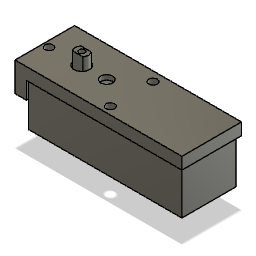
Moteur arduino v15 (Autodesk Fusion 360 design; units mm, degrees)
Autodesk Fusion 360 part; units mm, degrees
sketch "Esquisse1" plane through (0, 0, 0) normal (0, 1, 0) x (1, 0, 0)
  line L0 (0, 0) -> (64, 0)
  line L1 (64, 0) -> (64, 22.3)
  line L2 (64, 22.3) -> (0, 22.3)
  line L3 (0, 22.3) -> (0, 0)
  line L4 (0, 22.3) -> (10.9, 22.3)
  line L5 (10.9, 22.3) -> (10.9, 11.15)
  line L6 (10.9, 11.15) -> (0, 11.15)
  line L7 (0, 11.15) -> (0, 22.3)
  circle A0 centre (10.9, 11.15) radius 2.9
  line L8 (0, 22.3) -> (31.8, 22.3)
  line L9 (31.8, 22.3) -> (31.8, 20.1)
  line L10 (31.8, 20.1) -> (0, 20.1)
  line L11 (0, 20.1) -> (0, 22.3)
  circle A1 centre (31.8, 20.1) radius 1.8
  line L12 (0, 0) -> (31.8, 0)
  line L13 (31.8, 0) -> (31.8, 2.2)
  line L14 (31.8, 2.2) -> (0, 2.2)
  line L15 (0, 2.2) -> (0, 0)
  circle A2 centre (31.8, 2.2) radius 1.8
  dimension "d1" = 64
  dimension "d2" = 22.3
  dimension "d3" = 10.9
  dimension "d4" = 11.15
  dimension "d5" = 5.8
  dimension "d8" = 31.8
  dimension "d9" = 2.2
  dimension "d10" = 3.6
  dimension "d11" = 31.8
  dimension "d12" = 2.2
  dimension "d13" = 3.6
  constraint horizontal L0
  constraint vertical L1
  constraint horizontal L2
  constraint vertical L3
  constraint coincident L0.start L3.end
  constraint horizontal L4
  constraint vertical L5
  constraint horizontal L6
  constraint vertical L7
  constraint coincident L5.end L6.start
  constraint horizontal L8
  constraint vertical L9
  constraint horizontal L10
  constraint vertical L11
  constraint coincident L9.end L10.start
  constraint horizontal L12
  constraint vertical L13
  constraint horizontal L14
  constraint vertical L15
  constraint coincident L13.end L14.start
  measures "d1" distance of L0.start L0.end
  measures "d2" distance of L0.start L2.end
  measures "d3" distance of L2.end L4.end
  measures "d4" distance of L2.end L6.end
  measures "d5" diameter of A0
  measures "d8" distance of L2.end L8.end
  measures "d9" distance of L2.end L10.end
  measures "d10" diameter of A1
  measures "d11" distance of L0.start L12.end
  measures "d12" distance of L0.start L14.end
  measures "d13" diameter of A2
extrude "Extrusion1" add sketch "Esquisse1" along normal blind 19 contours L0 L3 L12 L13 L14 L15 A2 | L0 L1 L2 L3 L5 L6 A0 L9 L10 A1 L13 L14 A2 | L3 L5 L6 L7 A0 L10 | L2 L3 L4 L5 L7 L8 L10 L11 | L2 L5 L8 L9 L10 A1 makes body 1
sketch "Esquisse2" plane through (0, 0, 0) normal (-1, 0, 0) x (0, 0, 1)
  line L0 (-22.3, 0) -> (0, 0)
  line L1 (0, 0) -> (0, 19)
  line L2 (0, 19) -> (-22.3, 19)
  line L3 (-22.3, 19) -> (-22.3, 0)
  line L4 (-22.3, 19) -> (-13.3, 19)
  line L5 (-13.3, 19) -> (-13.3, 11)
  line L6 (-13.3, 11) -> (-22.3, 11)
  line L7 (-22.3, 11) -> (-22.3, 19)
  line L8 (-13.3, 11) -> (-8.3, 11)
  line L9 (-8.3, 11) -> (-8.3, 8)
  line L10 (-8.3, 8) -> (-13.3, 8)
  line L11 (-13.3, 8) -> (-13.3, 11)
  dimension "d14" = 9
  dimension "d15" = 8
  dimension "d16" = 5
  dimension "d17" = 3
  constraint horizontal L4
  constraint vertical L5
  constraint horizontal L6
  constraint vertical L7
  constraint coincident L2.end L3.start
  constraint horizontal L8
  constraint vertical L9
  constraint horizontal L10
  constraint vertical L11
  measures "d14" distance of L2.end L4.end
  measures "d15" distance of L2.end L6.end
  measures "d16" distance of L5.end L8.end
  measures "d17" distance of L5.end L10.end
extrude "Extrusion2" add sketch "Esquisse2" along normal blind 5 contours L8 L9 L10 L11 bodies 1
sketch "Esquisse3" plane through (0, 11, 0) normal (0, 1, 0) x (-1, 0, 0)
  line L0 (0, -8.3) -> (0, -13.3)
  line L1 (0, -13.3) -> (5, -13.3)
  line L2 (5, -13.3) -> (5, -8.3)
  line L3 (5, -8.3) -> (0, -8.3)
  circle A0 centre (2.5, -10.8) radius 1.7
  line L4 (0, -13.3) -> (1.2979, -12.0021)
  line L5 (3.7021, -9.5979) -> (5, -8.3)
  line L6 (5, -13.3) -> (3.7021, -12.0021)
  line L7 (1.2979, -9.5979) -> (0, -8.3)
  dimension "d20" = 3.4
  constraint coincident L0.end L1.start
  constraint coincident L2.end L3.start
  constraint coincident L1.end L2.start
  constraint coincident L0.start L3.end
  constraint coincident A0 L5.start
  constraint collinear L4 L5
  constraint coincident A0 L4.end
  constraint coincident A0 L6.end
  constraint coincident A0 L7.start
  constraint collinear L6 L7
  measures "d20" diameter of A0
extrude "Extrusion3" cut sketch "Esquisse3" against normal blind 5 contours A0 bodies 1
extrude "Extrusion4" add 1 faces at (0, 10, -19.3) along direction (-1, 0, 0) blind 0.2 on bodies 1 bodies 1
extrude "Extrusion5" add 1 faces at (-5, 10, -11.6333) along direction (-1, 0, 0) blind 0.2 on bodies 1 bodies 1
extrude "Extrusion6" add 1 faces at (-1.8667, 10, -8.3) along direction (0, 0, 1) blind 0.2 on bodies 1 bodies 1
extrude "Extrusion7" add 1 faces at (-3.5333, 10, -13.3) along direction (0, 0, -1) blind 0.2 on bodies 1 bodies 1
extrude "Extrusion8" add 1 faces at (42.6, 6.3333, -22.3) along direction (0, 0, -1) blind 0.2 on bodies 1 bodies 1
extrude "Extrusion9" add 1 faces at (42.6, 6.3333, 0) along direction (0, 0, 1) blind 0.2 on bodies 1 bodies 1
extrude "Extrusion10" add 1 faces at (53.7979, 19, -8.4455) along direction (0, 1, 0) blind 0.2 on bodies 1 bodies 1
extrude "Extrusion11" add 1 faces at (64, 6.4, -14.9333) along direction (1, 0, 0) blind 0.2 on bodies 1 bodies 1
copy_body "Corps->Comp1" bodies 1 removing the originals makes body 2 in component "Base"
sketch "Esquisse4" plane through (0, 0, 0) normal (0, 1, 0) x (1, 0, 0)
  circle A0 centre (-50, 5) radius 2.8
  dimension "d39" = 5.6
  measures "d39" diameter of A0
extrude "Extrusion12" add sketch "Esquisse4" along normal blind 37 separate body makes body 3
copy_body "Corps->Comp2" bodies 3 removing the originals makes body 4 in component "Axe"
sketch "Esquisse5" plane through (0, 28.2, 0) normal (0, 1, 0) x (-1, 0, 0)
  circle A0 centre (-10.9, -11.15) radius 2.8
sketch "Esquisse6" plane through (0, 28.2, 0) normal (0, 1, 0) x (-1, 0, 0)
  circle A0 centre (-10.9, -11.15) radius 2.8
  line L0 (-10.9, -11.15) -> (-13.7, -11.15)
  line L1 (-13.7, -11.15) -> (-8.097, -11.15)
  line L2 (-8.097, -11.15) -> (-13.697, -11.15)
  line L3 (-13.697, -11.15) -> (-13.697, -12.9)
  line L4 (-13.697, -12.9) -> (-8.097, -12.9)
  line L5 (-8.097, -12.9) -> (-8.097, -11.15)
  line L6 (-13.697, -12.9) -> (-8.097, -12.9)
  line L7 (-8.097, -12.9) -> (-8.097, -9.4)
  line L8 (-8.097, -9.4) -> (-13.697, -9.4)
  line L9 (-13.697, -9.4) -> (-13.697, -12.9)
  circle A1 centre (-10.9, -11.15) radius 1.2
  point P0 (-10.9, -11.15)
  dimension "d46" = 5.6
  dimension "d47" = 1.75
  dimension "d48" = 5.6
  dimension "d49" = 3.5
  dimension "d50" = 2.4
  constraint horizontal L0
  constraint coincident P0 A0.centre
  constraint coincident A0 L0.end
  constraint horizontal L2
  constraint vertical L3
  constraint horizontal L4
  constraint vertical L5
  constraint horizontal L6
  constraint vertical L7
  constraint horizontal L8
  constraint vertical L9
  constraint concentric A0 A1
  measures "d46" distance of L1.end L2.end
  measures "d47" distance of L1.end L4.end
  measures "d48" distance of L3.end L4.end
  measures "d49" distance of L3.end L8.end
  measures "d50" diameter of A1
extrude "Extrusion1'" cut sketch "Esquisse6" against normal blind 8 contours A0 L8 | A0 L4 L6 | L0 L1 L2 A1 | L0 L1 L2 A1 sketch seen with x (1, 0, 0) y (0, 1, 0) z (0, 0, 1) at (-60.9, 8.8, 6.15) bodies 4 in component "Axe"
sketch "Esquisse7" plane through (0, -8.8, 0) normal (0, -1, 0) x (1, 0, 0)
  circle A0 centre (10.9, -11.15) radius 2.8
  circle A1 centre (10.9, -11.15) radius 1.2
  line L0 (10.9, -11.15) -> (13.7, -11.15)
  line L1 (13.7, -11.15) -> (8.1, -11.15)
  line L2 (13.7, -11.15) -> (8.1, -11.15)
  line L3 (8.1, -11.15) -> (8.1, -9.4)
  line L4 (8.1, -9.4) -> (13.7, -9.4)
  line L5 (13.7, -9.4) -> (13.7, -11.15)
  line L6 (8.1, -9.4) -> (13.7, -9.4)
  line L7 (13.7, -9.4) -> (13.7, -12.9)
  line L8 (13.7, -12.9) -> (8.1, -12.9)
  line L9 (8.1, -12.9) -> (8.1, -9.4)
  dimension "d53" = 2.4
  dimension "d54" = 2.8
  dimension "d55" = 5.6
  dimension "d56" = 5.6
  dimension "d57" = 1.75
  dimension "d58" = 5.6
  dimension "d59" = 3.5
  constraint concentric A0 A1
  constraint coincident A0.centre A1.centre
  constraint horizontal L0
  constraint horizontal L2
  constraint vertical L3
  constraint horizontal L4
  constraint vertical L5
  constraint horizontal L6
  constraint vertical L7
  constraint horizontal L8
  constraint vertical L9
  measures "d53" diameter of A1
  measures "d54" distance of A0.centre L0.end
  measures "d55" distance of L0.end L1.end
  measures "d56" distance of L0.end L1.end
  measures "d57" distance of L0.end L4.end
  measures "d58" distance of L3.end L4.end
  measures "d59" distance of L3.end L8.end
extrude "Extrusion2'" cut sketch "Esquisse7" against normal blind 8 contours A0 L4 L6 | A0 L8 | A1 L0 L1 L2 | A1 L0 L1 L2 sketch seen with x (1, 0, 0) y (0, 1, 0) z (0, 0, 1) at (-60.9, 8.8, 6.15) bodies 4 in component "Axe"
sketch "Esquisse8" plane through (0, 19.2, 0) normal (0, 1, 0) x (-1, 0, 0)
  circle A0 centre (-31.8, -20.1) radius 1.8
  circle A1 centre (-31.8, -2.2) radius 1.8
  circle A2 centre (-10.9, -11.15) radius 2.9
  line L0 (-64.2, -22.5) -> (0.2, -22.5)
  line L1 (0.2, -22.5) -> (0.2, 0.2)
  line L2 (0.2, 0.2) -> (-64.2, 0.2)
  line L3 (-64.2, 0.2) -> (-64.2, -22.5)
  line L4 (-65, 1) -> (5, 1)
  line L5 (5, 1) -> (5, -24)
  line L6 (5, -24) -> (-65, -24)
  line L7 (-65, -24) -> (-65, 1)
  constraint horizontal L4
  constraint vertical L5
  constraint horizontal L6
  constraint vertical L7
extrude "Extrusion13" add sketch "Esquisse8" against normal blind 1 separate body contours L4 L5 L6 L7 makes body 5
sketch "Esquisse9" plane through (0, 19.2, 0) normal (0, 1, 0) x (-1, 0, 0)
  line L0 (-64.2, -22.5) -> (-64.2, 0.2)
  line L1 (-64.2, 0.2) -> (0.2, 0.2)
  line L2 (0.2, 0.2) -> (0.2, -22.5)
  line L3 (0.2, -22.5) -> (-64.2, -22.5)
  line L4 (-65, -24) -> (5, -24)
  line L5 (5, -24) -> (5, 1)
  line L6 (5, 1) -> (-65, 1)
  line L7 (-65, 1) -> (-65, -24)
  line L8 (5, -24) -> (-65, -24)
  line L9 (-65, -24) -> (-65, 1)
  line L10 (-65, 1) -> (5, 1)
  line L11 (5, 1) -> (5, -24)
  constraint horizontal L8
  constraint vertical L9
  constraint horizontal L10
  constraint vertical L11
  constraint coincident L6.end L7.start
  constraint coincident L4.end L5.start
extrude "Extrusion14" add sketch "Esquisse9" along normal blind 2 contours L0 L1 L2 L3 | L4 L5 L6 L7 L8 L9 L10 L11 bodies 5
sketch "Esquisse10" plane through (0, 0, 0) normal (0, -1, 0) x (1, 0, 0)
  circle A0 centre (31.8, -20.1) radius 1.8
  circle A1 centre (31.8, -2.2) radius 1.8
  circle A2 centre (10.9, -11.15) radius 2.9
  line L0 (64.2, 0.2) -> (-0.2, 0.2)
  line L1 (-0.2, 0.2) -> (-0.2, -22.5)
  line L2 (-0.2, -22.5) -> (64.2, -22.5)
  line L3 (64.2, -22.5) -> (64.2, 0.2)
  circle A3 centre (31.8, -2.2) radius 1.6
  circle A4 centre (31.8, -20.1) radius 1.6
  circle A5 centre (31.8, -2.2) radius 1.6
  circle A6 centre (10.9, -11.15) radius 3
  dimension "d66" = 3.2
  dimension "d67" = 3.2
  dimension "d68" = 6
  constraint concentric A1 A3
  constraint concentric A0 A4
  constraint concentric A3 A5
  constraint concentric A2 A6
  measures "d66" diameter of A4
  measures "d67" diameter of A5
  measures "d68" diameter of A6
extrude "Extrusion15" cut sketch "Esquisse10" against normal blind 22 contours A0 | A1 | A2 | A3 A5 | A4 | A6 bodies 5
sketch "Esquisse11" plane through (0, 8, 0) normal (0, -1, 0) x (1, 0, 0)
  line L0 (-0.2, -13.5) -> (-0.2, -8.1)
  line L1 (-0.2, -8.1) -> (-5.2, -8.1)
  line L2 (-5.2, -8.1) -> (-5.2, -13.5)
  line L3 (-5.2, -13.5) -> (-0.2, -13.5)
  circle A0 centre (-2.5, -10.8) radius 1.7
  circle A1 centre (-2.5, -10.8) radius 1.7
  dimension "d71" = 3.4
  constraint concentric A0 A1
  measures "d71" diameter of A1
extrude "Extrusion16" cut sketch "Esquisse11" against normal blind 15 contours A0 A1 bodies 5
sketch "Esquisse12" plane through (0, 18.2, 0) normal (0, -1, 0) x (1, 0, 0)
  circle A0 centre (-2.5, -10.8) radius 1.7
  line L0 (64.2, 0.2) -> (64.2, -22.5)
  line L1 (64.2, -22.5) -> (-0.2, -22.5)
  line L2 (-0.2, -22.5) -> (-0.2, 0.2)
  line L3 (-0.2, 0.2) -> (64.2, 0.2)
  line L4 (-5, -24) -> (65, -24)
  line L5 (65, -24) -> (65, 1)
  line L6 (65, 1) -> (-5, 1)
  line L7 (-5, 1) -> (-5, -24)
  line L8 (-5, -24) -> (-0.2, -24)
  line L9 (-0.2, -24) -> (-0.2, 1)
  line L10 (-0.2, 1) -> (-5, 1)
  line L11 (-5, 1) -> (-5, -24)
  constraint horizontal L8
  constraint vertical L9
  constraint horizontal L10
  constraint vertical L11
  constraint coincident L6 L9.end
  constraint coincident L4.start L7.end
extrude "Extrusion17" add sketch "Esquisse12" along normal blind 7.2 contours L2 L4 L6 L7 L8 L9 L10 L11 bodies 5
extrude "Extrusion18" cut 1 faces at (-2.635, 11, -20.1625) along direction (0, 1, 0) blind 0.5 on bodies 5 bodies 5
sketch "Esquisse13" plane through (0, 19.2, 0) normal (0, 1, 0) x (-1, 0, 0)
  circle A0 centre (-31.8, -2.2) radius 1.8
  circle A1 centre (-10.9, -11.15) radius 2.9
  circle A2 centre (-31.8, -20.1) radius 1.8
  line L0 (-64.2, -22.5) -> (0.2, -22.5)
  line L1 (0.2, -22.5) -> (0.2, 0.2)
  line L2 (0.2, 0.2) -> (-64.2, 0.2)
  line L3 (-64.2, 0.2) -> (-64.2, -22.5)
  line L4 (0.2, -22.5) -> (-21.3, -22.5)
  line L5 (-21.3, -22.5) -> (-21.3, -11.15)
  line L6 (-21.3, -11.15) -> (0.2, -11.15)
  line L7 (0.2, -11.15) -> (0.2, -22.5)
  circle A3 centre (-21.3, -11.15) radius 2.5
  dimension "d78" = 21.5
  dimension "d79" = 11.35
  dimension "d80" = 5
  constraint horizontal L4
  constraint vertical L5
  constraint horizontal L6
  constraint vertical L7
  constraint coincident L0.end L1.start
  constraint coincident L5.end L6.start
  measures "d78" distance of L0.end L4.end
  measures "d79" distance of L0.end L6.end
  measures "d80" diameter of A3
extrude "Extrusion1''" add sketch "Esquisse13" along normal blind 2 contours L5 L6 A3 | L5 L6 A3 bodies 2 in component "Base"
extrude "Extrusion19" cut 1 faces at (20.3768, 21.2, -11.8904) along direction (0, -1, 0) blind 2 on bodies 2 bodies 5
sketch "Esquisse14" plane through (0, 19.2, 0) normal (0, 1, 0) x (-1, 0, 0)
  circle A0 centre (-21.3, -11.15) radius 2.5
  circle A1 centre (-31.8, -2.2) radius 1.8
  circle A2 centre (-10.9, -11.15) radius 2.9
  circle A3 centre (-31.8, -20.1) radius 1.8
  line L0 (-64.2, -22.5) -> (0.2, -22.5)
  line L1 (0.2, -22.5) -> (0.2, 0.2)
  line L2 (0.2, 0.2) -> (-64.2, 0.2)
  line L3 (-64.2, 0.2) -> (-64.2, -22.5)
  line L4 (0.2, 0.2) -> (-37.3, 0.2)
  line L5 (-37.3, 0.2) -> (-37.3, -22.5)
  line L6 (-37.3, -22.5) -> (0.2, -22.5)
  line L7 (0.2, -22.5) -> (0.2, 0.2)
  dimension "d85" = 37.5
  constraint horizontal L4
  constraint vertical L5
  constraint horizontal L6
  constraint vertical L7
  constraint coincident L0 L5.end
  constraint coincident L1.end L2.start
  measures "d85" distance of L1.end L4.end
extrude "Extrusion2''" add sketch "Esquisse14" along normal blind 1.5 contours L0 L1 L2 L4 L5 L6 L7 bodies 2 in component "Base"
extrude "Extrusion20" cut 1 faces at (13.886, 20.7, -19.1971) along direction (0, -1, 0) blind 1.5 on bodies 2 bodies 5
extrude "Extrusion21" cut 1 faces at (55.2333, 19.2, -14.9333) along direction (0, 1, 0) blind 1.5 on bodies 5 bodies 5
extrude "Extrusion22" add 1 faces at (54.4646, 21.2, -14.0878) along direction (0, 1, 0) blind 2 on bodies 5 bodies 5
extrude "Extrusion23" add 1 faces at (-2.635, 11.5, -20.1625) along direction (0, -1, 0) blind 0.5 on bodies 5 bodies 5
sketch "Esquisse15" plane through (0, 23.2, 0) normal (0, 1, 0) x (-1, 0, 0)
  circle A0 centre (-21.3, -11.15) radius 2.5
  circle A1 centre (2.5, -10.8) radius 1.7
  circle A2 centre (-31.8, -20.1) radius 1.8
  circle A3 centre (-31.8, -2.2) radius 1.8
  circle A4 centre (-10.9, -11.15) radius 3
  line L0 (5, 1) -> (-65, 1)
  line L1 (-65, 1) -> (-65, -24)
  line L2 (-65, -24) -> (5, -24)
  line L3 (5, -24) -> (5, 1)
  circle A5 centre (-10.9, -11.15) radius 3.25
  dimension "d96" = 6.5
  constraint concentric A4 A5
  measures "d96" diameter of A5
extrude "Extrusion24" cut sketch "Esquisse15" against normal blind 2.5 contours A5 bodies 5
component "Base" placed x (1, 0, 0) y (0, 1, 0) z (0, 0, 1) at (0, 0, 0)
component "Axe" placed x (1, 0, 0) y (0, 1, 0) z (0, 0, 1) at (60.9, -8.8, -6.15)
equation "d3 = 8.3 mm + ( 5.2 / 2 ) * 1 mm"
equation "d9 = 0.6 mm + 1.6 mm"
equation "d47 = ( 3.5 / 2 ) * 1 mm"
equation "d54 = ( 5.6 / 2 ) * 1 mm"
equation "d57 = ( 3.5 / 2 ) * 1 mm"
equation "d78 = 24 mm - 2 mm - 0.5 mm"
equation "d79 = ( 22.7 / 2 ) * 1 mm"
